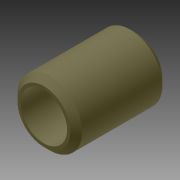
# Autodesk Inventor part: D-8597
Saved by Autodesk Inventor 2014 (Build 180170000, 170)
## iProperties
Created: 2014-01-19
Part Number: D-8597
Material: Generic
Catalog Web Link: www.cadenas.de
Description: Bushing-Original Line - Standard Air Cylinders
Vendor: BIMBA
Document SubType Name: Standard Catalog Part
Designer: Michael
Manufacturer: BIMBA
Density: 1 g/cm^3
Appearance: RGB(181.04999452829415,165.74999392032569,66.29999756813130)
Category: PARTsolutions
Company: BIMBA
Title: D-8597
Author: Cadenas PARTsolutions
Comments: Original Line - Standard Air Cylinders
PSOL_IDENT_0: {$CADENAS_DATA\23d-libs\bimba\bimba\bimba_imperial\bimba_full_line\original_line_cylinders\standard_
PSOL_IDENT_1: air_cylinders\bushing.prj},155 {VTYP=3D},{NB=D-8597},{LINA=D-8597},{NN=Bushing},{DATE=13.09.2012 05:
PSOL_IDENT_2: 23:39},{GEOMDATE=10.09.2012 00:00:00},{VERSION=},{LINEID=20},{LINESUBID=-1},{WBVAR=}  {NB=D-8597},{L
PSOL_IDENT_3: INA=D-8597},{KT=DUMMY},{PN=D-8597},{ID=0.1570},{OD=0.2185},{L=0.3120},{C=0.0200}
CNS_NN: Bushing
CNS_NT: Original Line - Standard Air Cylinders
CNS_NB: D-8597
CNS_NBSYN: $PN.
CNS_LINA: D-8597
CNS_PN: D-8597
CNS_ID: 0.1570
CNS_OD: 0.2185
CNS_L: 0.3120
CNS_C: 0.0200
SUPPLIER: BIMBA
ARTICLENO: D-8597
BOMINFO: D-8597
CREATOR: CADENAS GmbH
Autodesk Inventor part; units mm, degrees
ref_plane "YZ Plane" through (0, 0, 0) normal (1, 0, 0) x (0, 1, 0)
ref_plane "XZ Plane" through (0, 0, 0) normal (0, 1, 0) x (-1, 0, 0)
ref_plane "XY Plane" through (0, 0, 0) normal (0, 0, 1) x (1, 0, 0)
sketch "Sketch_1" plane through (0, 0, 0) normal (1, 0, 0) x (0, 1, 0)
  line L0 (0, -3.9624) -> (0, 3.9624)
  line L1 (2.2669, 3.9624) -> (1.9939, 3.9624)
  line L2 (1.9939, 3.9624) -> (1.9939, -3.9624)
  line L3 (1.9939, -3.9624) -> (2.2669, -3.9624)
  line L4 (2.2669, -3.9624) -> (2.775, -3.4544)
  line L5 (2.775, -3.4544) -> (2.775, 3.4544)
  line L6 (2.775, 3.4544) -> (2.2669, 3.9624)
  constraints: 14 end point
revolve "Revolution1" add sketch "Sketch_1" angle 360 about axis through (0, 0, -3.9624) along (0, 0, -1)
ref_plane "bushing_XY" through (0, 0, 0) normal (0, 0, 1) x (1, 0, 0)
ref_plane "bushing_YZ" through (0, 0, 0) normal (1, 0, 0) x (0, 1, 0)
ref_plane "bushing_ZX" through (0, 0, 0) normal (0, 1, 0) x (0, 0, 1)
ref_plane "id1_XY" through (-1.9939, 0, 0) normal (0, 0, 1) x (1, 0, 0)
ref_plane "id1_YZ" through (-1.9939, 0, 0) normal (1, 0, 0) x (0, 1, 0)
ref_plane "id1_ZX" through (-1.9939, 0, 0) normal (0, 1, 0) x (0, 0, 1)
ref_plane "id2_XY" through (1.9939, 0, 0) normal (0, 0, 1) x (1, 0, 0)
ref_plane "id2_YZ" through (1.9939, 0, 0) normal (1, 0, 0) x (0, 1, 0)
ref_plane "id2_ZX" through (1.9939, 0, 0) normal (0, 1, 0) x (0, 0, 1)
ref_plane "id3_XY" through (0, 0, -3.9624) normal (0, 0, -1) x (0, 1, 0)
ref_plane "id3_YZ" through (0, 0, -3.9624) normal (0, 1, 0) x (1, 0, 0)
ref_plane "id3_ZX" through (0, 0, -3.9624) normal (1, 0, 0) x (0, 0, -1)
ref_plane "id4_XY" through (0, 0, 3.9624) normal (0, 0, 1) x (0, 1, 0)
ref_plane "id4_YZ" through (0, 0, 3.9624) normal (0, 1, 0) x (-1, 0, 0)
ref_plane "id4_ZX" through (0, 0, 3.9624) normal (-1, 0, 0) x (0, 0, 1)
body "Solid1"
